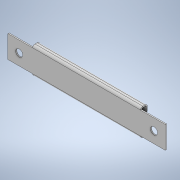
# Autodesk Inventor part: Suporte lateral da bateria
Saved by Autodesk Inventor 2021 (Build 250183000, 183)
## iProperties
Created: 2021-12-07
Part Number: Suporte lateral da bateria
Material: Generic
Document SubType Name: Sheet Metal
Designer: Matheus
Density: 1 g/cm^3
Sheet Metal Rule: Default_mm
Appearance: Default
Author: Matheus
Autodesk Inventor part; units mm, degrees
ref_plane "YZ Plane" through (0, 0, 0) normal (1, 0, 0) x (0, 1, 0)
ref_plane "XZ Plane" through (0, 0, 0) normal (0, 1, 0) x (-1, 0, 0)
ref_plane "XY Plane" through (0, 0, 0) normal (0, 0, 1) x (1, 0, 0)
sketch "Sketch1" plane through (0, 0, 0) normal (0, 0, 1) x (1, 0, 0)
  line L0 (35, 5) -> (35, -5)
  line L1 (-35, -5) -> (-35, 5)
  line L2 (-49, 0) -> (49, 0) construction
  line L3 (0, -8.4) -> (0, 8.4) construction
  line L4 (24, 5) -> (24, 6)
  line L5 (24, 6) -> (-24, 6)
  line L6 (-24, 6) -> (-24, 5)
  line L7 (24, -5) -> (24, -6)
  line L8 (24, -6) -> (-24, -6)
  line L9 (-24, -6) -> (-24, -5)
  line L10 (-35, 5) -> (-24, 5)
  line L11 (24, 5) -> (35, 5)
  line L12 (35, -5) -> (24, -5)
  line L13 (-24, -5) -> (-35, -5)
  point P0 (0, 0)
  dimension "d0" = 10
  dimension "d1" = 70
  dimension "d46" = 48
  dimension "d51" = 1
  measures "d0" distance of L1.start L1.end
  measures "d1" distance of L1.end L0.start
  measures "d46" distance of L4.end L5.end
  measures "d51" distance between parallel lines of L10 L5
extrude "Plate1" add sketch "Sketch1" along normal mid plane 0.5
sketch "Sketch5" plane through (0, 0, -0.25) normal (0, 0, -1) x (-1, 0, 0)
  line L0 (0, -8.4) -> (0, 8.4) construction
  line L1 (49, 0) -> (-49, 0) construction
  point P0 (0, 0)
  point P1 (-30, 0)
  point P2 (30, 0)
  dimension "d26" = 60
  constraints: 2 point on line, 1 symmetric about line
  measures "d26" distance of point (30, 0) point (-30, 0)
hole "Hole1" at (30, 0, -0.25) at (-30, 0, -0.25) direction (0, 0, 1) diameter 3.2 end through all
sketch "Sketch8" plane through (24, 5.5, 0.25) normal (0, 1, 0) x (-1, 0, 0)
  line L0 (48, 0) -> (0, 0)
  line L1 (0, 0) -> (0, -3)
  line L2 (0, -3) -> (48, -3)
  line L3 (48, -3) -> (48, 0)
  constraints: 6 end point, 1 horizontal, 1 perpendicular, 1 vertical
edge flange "Flange4" height 3 angle 90 thickness 0.5 bend radius 0.5 thickness toward (0, 1, 0) relief straight relief width 0.5 relief depth 0.25 corner gap 0.5 corner form 0 edges at (0, 6, -0.25) (0, -6, -0.25) wall of the first edge with corners at (-24, 5.5, 0.25) (24, 5.5, 0.25) (24, 5.5, -2.75) (-24, 5.5, -2.75)
bend "Bend4"
corner "Corner4"
sketch "Sketch9" plane through (24, 6, -2.25) normal (0, 0, -1) x (-1, 0, 0)
  line L0 (48, 0) -> (0, 0)
  line L1 (0, 0) -> (0, -3)
  line L2 (0, -3) -> (48, -3)
  line L3 (48, -3) -> (48, 0)
  constraints: 6 end point, 1 horizontal, 1 perpendicular, 1 vertical
edge flange "Flange5" height 3 angle 90 thickness 0.5 bend radius 0.5 thickness toward (0, 0, -1) relief straight relief width 0.5 relief depth 0.25 corner gap 0.5 corner form 0 edges at (0, 5.5, -2.75) (0, -5.5, -2.75) wall of the first edge with corners at (-24, 6, -2.25) (24, 6, -2.25) (24, 3, -2.25) (-24, 3, -2.25)
bend "Bend5"
corner "Corner5"
equation "\"d32\" = Thickness"
equation "\"d2\" = Thickness"
equation "\"d52\" = BendReliefWidth"
equation "\"d53\" = BendReliefDepth"
equation "\"d54\" = MinimumRemnant"
equation "\"d55\" = TransitionRadius"
equation "\"d58\" = BendRadius"
equation "\"d59\" = CornerReliefSize"
equation "\"d60\" = GapSize"
equation "\"d61\" = JacobiRadiusSize"
equation "\"d62\" = BendReliefWidth"
equation "\"d63\" = BendReliefDepth"
equation "\"d64\" = MinimumRemnant"
equation "\"d65\" = TransitionRadius"
equation "\"d68\" = BendRadius"
equation "\"d69\" = CornerReliefSize"
equation "\"d70\" = GapSize"
equation "\"d71\" = JacobiRadiusSize"
equation "\"BendRadius\" = Thickness"
equation "\"BendReliefWidth\" = Thickness"
equation "\"BendReliefDepth\" = 0.5 * Thickness"
equation "\"CornerReliefSize\" = 4 * Thickness"
equation "\"MinimumRemnant\" = 2 * Thickness"
equation "\"TransitionRadius\" = BendRadius"
equation "\"JacobiRadiusSize\" = BendRadius"
equation "\"GapSize\" = Thickness"
equation "\"Thickness\" = 0.5"
body "Solid1"
